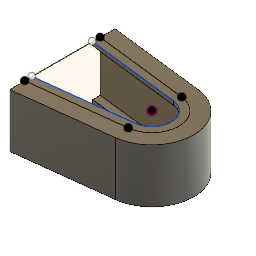
sjointjoint (Autodesk Fusion 360 design; units mm, degrees)
Autodesk Fusion 360 part; units mm, degrees
sketch "スケッチ1" plane through (0, 0, 0) normal (0, 1, 0) x (1, 0, 0)
  circle A0 centre (0, 0) radius 1.25
  circle A1 centre (0, 0) radius 2.5
  circle A2 centre (14.5, 0) radius 0.5
  circle A3 centre (4.5, 0) radius 0.5
  circle A4 centre (6.5, 0) radius 0.5
  circle A5 centre (8.5, 0) radius 0.5
  circle A6 centre (10.5, 0) radius 0.5
  circle A7 centre (12.5, 0) radius 0.5
  line L0 (0, 10) -> (0, -8)
  circle A8 centre (-8.5, 0) radius 0.5
  circle A9 centre (-14.5, 0) radius 0.5
  circle A10 centre (-10.5, 0) radius 0.5
  circle A11 centre (-12.5, 0) radius 0.5
  circle A12 centre (-4.5, 0) radius 0.5
  circle A13 centre (-6.5, 0) radius 0.5
  line L1 (-0.4103, 3.4759) -> (-14.711, 1.7876)
  line L2 (-21, 0) -> (22, 0)
  line L3 (0.4103, 3.4759) -> (14.711, 1.7876)
  line L4 (-0.4103, -3.4759) -> (-14.711, -1.7876)
  line L5 (0.4103, -3.4759) -> (14.711, -1.7876)
  arc A14 (-12.7525, -0.4316) -> (-12.7525, 0.4316) centre (-14.5, 0) ccw
  arc A15 (-14.711, 1.7876) -> (-14.711, -1.7876) centre (-14.5, 0) ccw
  arc A16 (14.711, -1.7876) -> (14.711, 1.7876) centre (14.5, 0) ccw
  arc A17 (12.7525, 0.4316) -> (12.7525, -0.4316) centre (14.5, 0) ccw
  arc A18 (-0.4103, -3.4759) -> (0.4103, -3.4759) centre (0, 0) ccw
  arc A19 (0.4103, 3.4759) -> (-0.4103, 3.4759) centre (0, 0) ccw
  dimension "d1" = 2.5
  dimension "d2" = 5
  dimension "d4" = 3.6
  dimension "d7" = 2
  dimension "d8" = 0
  constraint coincident A0.centre A1.centre
  constraint concentric A0 A1
  constraint concentric A2 A16
  constraint vertical L0
  constraint symmetric A2 L0 A9
  constraint symmetric L0 A14 A16
  constraint symmetric A3 L0 A12
  constraint symmetric A4 L0 A13
  constraint symmetric A5 L0 A8
  constraint symmetric A6 L0 A10
  constraint symmetric A7 L0 A11
  constraint tangent L1 A18
  constraint coincident L1.end A14
  constraint tangent L1 A14
  constraint horizontal L2
  constraint symmetric L0 L1.start L3.start
  constraint symmetric L0 L1.end L3.end
  constraint symmetric L1.start L2 L4.start
  constraint symmetric L1.end L2 L4.end
  constraint symmetric L2 L3.start L5.start
  constraint symmetric L2 L3.end L5.end
  constraint coincident A11 A14.start
  constraint coincident A11 A14.end
  constraint concentric A14 A15
  constraint coincident A7 A17.end
  constraint coincident A7 A17.start
  constraint concentric A16 A17
  constraint concentric A18 A19
  measures "d1" diameter of A0
  measures "d2" diameter of A1
  measures "d4" diameter of A16
extrude "押し出し1" add sketch "スケッチ1" along normal blind 1.5 contours A0 L0 L2 | A0 A1 L0 L2 | A0 A1 L0 L2 | A0 L0 L2 | A0 L0 L2 | A0 A1 L0 L2 | A0 A1 L0 L2 | A0 L0 L2 | A1 A2 A3 A4 A5 A6 A7 L0 L2 L5 A16 A18 | A1 A2 A3 A4 A5 A6 A7 L0 L2 L3 A16 A19 | A1 L0 A8 A9 A10 A11 A12 A13 L1 L2 A15 A19 | A1 L0 A8 A9 A10 A11 A12 A13 L2 L4 A15 A18 makes body 1
sketch "スケッチ2" plane through (0, 1.5, 0) normal (0, 1, 0) x (-1, 0, 0)
  circle A0 centre (-14.5, 0) radius 0.5
  circle A1 centre (4.5, 0) radius 0.5
  circle A2 centre (-10.5, 0) radius 0.5
  circle A3 centre (12.5, 0) radius 0.5
  circle A4 centre (-8.5, 0) radius 0.5
  circle A5 centre (14.5, 0) radius 0.5
  circle A6 centre (10.5, 0) radius 0.5
  circle A7 centre (-12.5, 0) radius 0.5
  circle A8 centre (-6.5, 0) radius 0.5
  circle A9 centre (8.5, 0) radius 0.5
  circle A10 centre (-4.5, 0) radius 0.5
  circle A11 centre (6.5, 0) radius 0.5
  arc A12 (0.4103, 3.4759) -> (-0.4103, 3.4759) centre (0, 0) ccw
  line L0 (-0.4103, 3.4759) -> (-14.711, 1.7876)
  arc A13 (-14.711, 1.7876) -> (-14.711, -1.7876) centre (-14.5, 0) ccw
  line L1 (-14.711, -1.7876) -> (-0.4103, -3.4759)
  arc A14 (-0.4103, -3.4759) -> (0.4103, -3.4759) centre (0, 0) ccw
  line L2 (0.4103, -3.4759) -> (14.711, -1.7876)
  arc A15 (14.711, -1.7876) -> (14.711, 1.7876) centre (14.5, 0) ccw
  line L3 (14.711, 1.7876) -> (0.4103, 3.4759)
  circle A16 centre (0, 0) radius 3.1
  dimension "d11" = 6.2
  constraint coincident A12.centre A14.centre
  measures "d11" diameter of A16
extrude "押し出し2" add sketch "スケッチ2" along normal blind 5 contours A16 bodies 1
sketch "スケッチ3" plane through (0, 6.5, 0) normal (0, 1, 0) x (-1, 0, 0)
  circle A0 centre (0, 0) radius 3.1
  circle A1 centre (0, 0) radius 4
  dimension "d14" = 8
  constraint coincident A0.centre A1.centre
  measures "d14" diameter of A1
delete_face "面を削除1" 1 faces at (-3.0961, 4.8333, -0.1545) on bodies 1
sketch "スケッチ5" plane through (0, 0, 0) normal (0, 1, 0) x (1, 0, 0)
  circle A0 centre (0, 0) radius 4
  circle A1 centre (0, 0) radius 3.25
  dimension "d17" = 8
  dimension "d18" = 6.5
  constraint coincident A0.centre A1.centre
  constraint concentric A0 A1
  measures "d17" diameter of A0
  measures "d18" diameter of A1
extrude "押し出し4" add sketch "スケッチ5" along normal blind 6.5 bodies 1
copy_body "ボディのコピーと貼り付け1" bodies 1 makes body 2
mirror "ミラー1" about plane through (0, 0, 0) normal (0, 1, 0) of bodies 1 makes body 3
sketch "スケッチ6" plane through (0, 0, 0) normal (0, 1, 0) x (1, 0, 0)
  line L0 (2.3335, -3.2488) -> (14.711, -1.7876)
  arc A0 (14.711, -1.7876) -> (14.711, 1.7876) centre (14.5, 0) ccw
  line L1 (14.711, 1.7876) -> (2.3335, 3.2488)
  line L2 (2.4507, -4.2419) -> (14.8283, -2.7807)
  arc A1 (14.8283, -2.7807) -> (14.8283, 2.7807) centre (14.5, 0) ccw
  line L3 (14.8283, 2.7807) -> (2.4507, 4.2419)
  line L4 (0.9119, 6.5268) -> (8.5223, 6.5268)
  line L5 (8.5223, 6.5268) -> (8.5223, -5.886)
  line L6 (8.5223, -5.886) -> (0.9119, -5.886)
  line L7 (0.9119, -5.886) -> (0.9119, 6.5268)
  point P0 (8.5223, 3.5252)
  point P1 (8.5223, -3.5252)
  dimension "d22" = 1
  constraint coincident L3 P0
  constraint coincident L2 P1
  constraint horizontal L4
  constraint vertical L5
  constraint horizontal L6
  constraint vertical L7
extrude "押し出し5" add sketch "スケッチ6" along normal mid plane 3.6 contours L0 A0 L1 L2 A1 L3 L5 bodies 1 2 3
sketch "スケッチ7" plane through (0, 1.8, 0) normal (0, 1, 0) x (-1, 0, 0)
  line L0 (-8.5223, 2.5182) -> (-8.5223, 3.5252)
  line L1 (-8.5223, 3.5252) -> (-14.8283, 2.7807)
  arc A0 (-14.8283, 2.7807) -> (-14.8283, -2.7807) centre (-14.5, 0) ccw
  line L2 (-14.8283, -2.7807) -> (-8.5223, -3.5252)
  line L3 (-8.5223, -3.5252) -> (-8.5223, -2.5182)
  line L4 (-8.5223, -2.5182) -> (-14.711, -1.7876)
  arc A1 (-14.711, 1.7876) -> (-14.711, -1.7876) centre (-14.5, 0) ccw
  line L5 (-14.711, 1.7876) -> (-8.5223, 2.5182)
  line L6 (-8.5223, -2.5182) -> (-14.711, -1.7876)
  arc A2 (-14.711, 1.7876) -> (-14.711, -1.7876) centre (-14.5, 0) ccw
  line L7 (-14.711, 1.7876) -> (-8.5223, 2.5182)
  line L8 (-8.503, -2.017) -> (-14.6524, -1.291)
  arc A3 (-14.6524, 1.291) -> (-14.6524, -1.291) centre (-14.5, 0) ccw
  line L9 (-14.6524, 1.291) -> (-8.503, 2.017)
  line L10 (-8.5223, -2.5182) -> (-14.711, -1.7876)
  line L11 (-14.711, 1.7876) -> (-8.5223, 2.5182)
  arc A4 (-14.711, 1.7876) -> (-14.711, -1.7876) centre (-14.5, 0) ccw
  line L12 (-8.5223, -2.5182) -> (-8.5223, 2.5182)
  constraint parallel L6 L8
  constraint concentric A2 A3
  constraint parallel L7 L9
  constraint tangent A3 L9
  constraint tangent L8 A3
  constraint coincident L3.end L4.start
  constraint coincident L4.end A1.end
  constraint coincident A1.start L5.start
  constraint coincident L0.start L5.end
  constraint concentric A2 A4
  constraint coincident L4.end A4
extrude "押し出し6" add sketch "スケッチ7" against normal blind 0.25 contours L4 A1 L5 L6 A2 L7 L8 A3 L9 L10 L11 A4 L12 bodies 1
extrude "押し出し7" add sketch "スケッチ7" against normal blind 1.8 separate body contours L0 L1 A0 L2 L3 L4 A1 L5 L6 A2 L7 L10 L11 A4 makes body 4
extrude "押し出し8" add sketch "スケッチ7" against normal blind 0.25 contours L4 A1 L5 L6 A2 L7 L8 A3 L9 L10 L11 A4 L12 bodies 4
mirror "ミラー2" about plane through (0, 0, 0) normal (0, 1, 0) of bodies 4 makes body 5
combine "結合1" operation add target body 4 tool bodies 5
extrude "押し出し3" [rolled back] along distance -6.5 taper angle 0
sketch "スケッチ4" plane through (0, 0, 0) normal (0, 1, 0) x (1, 0, 0)
hidden bodies 1
